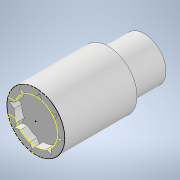
# Autodesk Inventor part: handle_base3
Saved by Autodesk Inventor 2021 (Build 250183000, 183)
## iProperties
Created: 2021-07-05
Part Number: handle_base3
Material: Generic
Document SubType Name: Modeling
Designer: teh18
Density: 1 g/cm^3
Appearance: Default
Author: teh18
Autodesk Inventor part; units mm, degrees
ref_plane "YZ Plane" through (0, 0, 0) normal (1, 0, 0) x (0, 1, 0)
ref_plane "XZ Plane" through (0, 0, 0) normal (0, 1, 0) x (-1, 0, 0)
ref_plane "XY Plane" through (0, 0, 0) normal (0, 0, 1) x (1, 0, 0)
sketch "Sketch1" plane through (0, 0, 0) normal (0, 0, 1) x (1, 0, 0)
  circle A0 centre (0, 0) radius 6
  circle A1 centre (0, 0) radius 20 projected
  circle A2 centre (0, 0) radius 5 projected
  arc A3 (6.0947, -0.2544) -> (5.2397, 3.1233) centre (0, 0) ccw projected
  arc A4 (4.1297, -4.4895) -> (5.9136, -1.4965) centre (0, 0) ccw projected
  arc A5 (-0.2544, -6.0947) -> (3.1233, -5.2397) centre (0, 0) ccw projected
  arc A6 (-4.4895, -4.1297) -> (-1.4965, -5.9136) centre (0, 0) ccw projected
  arc A7 (-6.0947, 0.2544) -> (-5.2397, -3.1233) centre (0, 0) ccw projected
  arc A8 (-4.1297, 4.4895) -> (-5.9136, 1.4965) centre (0, 0) ccw projected
  arc A9 (0.2544, 6.0947) -> (-3.1233, 5.2397) centre (0, 0) ccw projected
  arc A10 (4.4895, 4.1297) -> (1.4965, 5.9136) centre (0, 0) ccw projected
  line L0 (5.7362, 4.2762) -> (5.2397, 3.1233) projected
  line L1 (6.0947, -0.2544) -> (7.0798, -1.0323) projected
  line L2 (7.0798, -1.0323) -> (5.9136, -1.4965) projected
  line L3 (4.1297, -4.4895) -> (4.2762, -5.7362) projected
  line L4 (4.2762, -5.7362) -> (3.1233, -5.2397) projected
  line L5 (-0.2544, -6.0947) -> (-1.0323, -7.0798) projected
  line L6 (-1.0323, -7.0798) -> (-1.4965, -5.9136) projected
  line L7 (-4.4895, -4.1297) -> (-5.7362, -4.2762) projected
  line L8 (-5.7362, -4.2762) -> (-5.2397, -3.1233) projected
  line L9 (-6.0947, 0.2544) -> (-7.0798, 1.0323) projected
  line L10 (-7.0798, 1.0323) -> (-5.9136, 1.4965) projected
  line L11 (-4.1297, 4.4895) -> (-4.2762, 5.7362) projected
  line L12 (-4.2762, 5.7362) -> (-3.1233, 5.2397) projected
  line L13 (0.2544, 6.0947) -> (1.0323, 7.0798) projected
  line L14 (1.0323, 7.0798) -> (1.4965, 5.9136) projected
  line L15 (4.4895, 4.1297) -> (5.7362, 4.2762) projected
  line L16 (4.1567, -5.5758) -> (4.0244, -4.4502)
  arc A11 (4.0244, -4.4502) -> (5.8289, -1.4226) centre (0, 0) ccw
  line L17 (5.8289, -1.4226) -> (6.8819, -1.0035)
  line L18 (6.8819, -1.0035) -> (5.9924, -0.3011)
  arc A12 (5.9924, -0.3011) -> (5.1276, 3.1157) centre (0, 0) ccw
  line L19 (5.1276, 3.1157) -> (5.5758, 4.1567)
  line L20 (5.5758, 4.1567) -> (4.4502, 4.0244)
  arc A13 (4.4502, 4.0244) -> (1.4226, 5.8289) centre (0, 0) ccw
  line L21 (1.4226, 5.8289) -> (1.0035, 6.8819)
  line L22 (1.0035, 6.8819) -> (0.3011, 5.9924)
  arc A14 (0.3011, 5.9924) -> (-3.1157, 5.1276) centre (0, 0) ccw
  line L23 (-3.1157, 5.1276) -> (-4.1567, 5.5758)
  line L24 (-4.1567, 5.5758) -> (-4.0244, 4.4502)
  arc A15 (-4.0244, 4.4502) -> (-5.8289, 1.4226) centre (0, 0) ccw
  line L25 (-5.8289, 1.4226) -> (-6.8819, 1.0035)
  line L26 (-6.8819, 1.0035) -> (-5.9924, 0.3011)
  arc A16 (-5.9924, 0.3011) -> (-5.1276, -3.1157) centre (0, 0) ccw
  line L27 (-5.1276, -3.1157) -> (-5.5758, -4.1567)
  line L28 (-5.5758, -4.1567) -> (-4.4502, -4.0244)
  arc A17 (-4.4502, -4.0244) -> (-1.4226, -5.8289) centre (0, 0) ccw
  line L29 (-1.4226, -5.8289) -> (-1.0035, -6.8819)
  line L30 (-1.0035, -6.8819) -> (-0.3011, -5.9924)
  arc A18 (-0.3011, -5.9924) -> (3.1157, -5.1276) centre (0, 0) ccw
  line L31 (3.1157, -5.1276) -> (4.1567, -5.5758)
  point P0 (0, 0)
  point P1 (0, 0)
  point P2 (5.8289, -1.4226)
  point P3 (3.1157, -5.1276)
  point P4 (-1.4226, -5.8289)
  point P5 (-5.1276, -3.1157)
  point P6 (-5.8289, 1.4226)
  point P7 (-3.1157, 5.1276)
  point P8 (1.4226, 5.8289)
  point P9 (5.1276, 3.1157)
  dimension "d0" = 0.1
  dimension "d14" = 0.1
  constraints: 32 end point, 16 point on circle, 9 centre point, 23 other
  measures "d0" radial gap between concentric circles of A3 A0
  measures "d14" distance between parallel lines of L3 L16
extrude "Extrusion1" add sketch "Sketch1" against normal blind 10 contours A0 | A0 L20 L19 | L18 L17 A0 | A0 L22 L21 | L16 L31 A0 | A0 L24 L23 | L30 L29 A0 | A0 L26 L25 | L28 L27 A0
sketch "Sketch2" plane through (0, 0, 0) normal (0, 0, 1) x (1, 0, 0)
  circle A0 centre (0, 0) radius 6.1 projected
  arc A1 (5.9924, -0.3011) -> (5.1276, 3.1157) centre (0, 0) ccw projected
  circle A2 centre (0, 0) radius 18
  circle A3 centre (0, 0) radius 20 projected
  point P0 (0, 0)
  constraints: 1 centre point
extrude "Extrusion2" add sketch "Sketch2" along normal blind 20 contours A0 | A2
sketch "Sketch6" plane through (0, 0, 20) normal (0, 0, 1) x (0, -1, 0)
  circle A0 centre (0, 0) radius 8 projected
  arc A1 (-4.2421, -4.1006) -> (-1.5887, -5.6821) centre (0, 0) ccw projected
  line L0 (-1.5887, -5.6821) -> (-1.0323, -7.0798) projected
  line L1 (-1.0323, -7.0798) -> (-0.1, -5.8992) projected
  arc A2 (-0.1, -5.8992) -> (2.8945, -5.1412) centre (0, 0) ccw projected
  line L2 (2.8945, -5.1412) -> (4.2762, -5.7362) projected
  line L3 (4.2762, -5.7362) -> (4.1006, -4.2421) projected
  arc A3 (4.1006, -4.2421) -> (5.6821, -1.5887) centre (0, 0) ccw projected
  line L4 (5.6821, -1.5887) -> (7.0798, -1.0323) projected
  line L5 (7.0798, -1.0323) -> (5.8992, -0.1) projected
  arc A4 (5.8992, -0.1) -> (5.1412, 2.8945) centre (0, 0) ccw projected
  line L6 (5.1412, 2.8945) -> (5.7362, 4.2762) projected
  line L7 (5.7362, 4.2762) -> (4.2421, 4.1006) projected
  arc A5 (4.2421, 4.1006) -> (1.5887, 5.6821) centre (0, 0) ccw projected
  line L8 (1.5887, 5.6821) -> (1.0323, 7.0798) projected
  line L9 (1.0323, 7.0798) -> (0.1, 5.8992) projected
  arc A6 (0.1, 5.8992) -> (-2.8945, 5.1412) centre (0, 0) ccw projected
  line L10 (-2.8945, 5.1412) -> (-4.2762, 5.7362) projected
  line L11 (-4.2762, 5.7362) -> (-4.1006, 4.2421) projected
  arc A7 (-4.1006, 4.2421) -> (-5.6821, 1.5887) centre (0, 0) ccw projected
  line L12 (-5.6821, 1.5887) -> (-7.0798, 1.0323) projected
  line L13 (-7.0798, 1.0323) -> (-5.8992, 0.1) projected
  arc A8 (-5.8992, 0.1) -> (-5.1412, -2.8945) centre (0, 0) ccw projected
  line L14 (-5.1412, -2.8945) -> (-5.7362, -4.2762) projected
  line L15 (-5.7362, -4.2762) -> (-4.2421, -4.1006) projected
  arc A9 (4.2796, 4.2066) -> (1.664, 5.7655) centre (0, 0) ccw
  line L16 (4.2796, 4.2066) -> (5.8979, 4.3968)
  line L17 (5.8979, 4.3968) -> (5.2535, 2.9002)
  arc A10 (6.0006, -0.0517) -> (5.2535, 2.9002) centre (0, 0) ccw
  line L18 (6.0006, -0.0517) -> (7.2794, -1.0614)
  line L19 (7.2794, -1.0614) -> (5.7655, -1.664)
  arc A11 (4.2066, -4.2796) -> (5.7655, -1.664) centre (0, 0) ccw
  line L20 (4.2066, -4.2796) -> (4.3968, -5.8979)
  line L21 (4.3968, -5.8979) -> (2.9002, -5.2535)
  arc A12 (-0.0517, -6.0006) -> (2.9002, -5.2535) centre (0, 0) ccw
  line L22 (-0.0517, -6.0006) -> (-1.0614, -7.2794)
  line L23 (-1.0614, -7.2794) -> (-1.664, -5.7655)
  arc A13 (-4.2796, -4.2066) -> (-1.664, -5.7655) centre (0, 0) ccw
  line L24 (-4.2796, -4.2066) -> (-5.8979, -4.3968)
  line L25 (-5.8979, -4.3968) -> (-5.2535, -2.9002)
  arc A14 (-6.0006, 0.0517) -> (-5.2535, -2.9002) centre (0, 0) ccw
  line L26 (-6.0006, 0.0517) -> (-7.2794, 1.0614)
  line L27 (-7.2794, 1.0614) -> (-5.7655, 1.664)
  arc A15 (-4.2066, 4.2796) -> (-5.7655, 1.664) centre (0, 0) ccw
  line L28 (-4.2066, 4.2796) -> (-4.3968, 5.8979)
  line L29 (-4.3968, 5.8979) -> (-2.9002, 5.2535)
  arc A16 (0.0517, 6.0006) -> (-2.9002, 5.2535) centre (0, 0) ccw
  line L30 (0.0517, 6.0006) -> (1.0614, 7.2794)
  line L31 (1.0614, 7.2794) -> (1.664, 5.7655)
  point P0 (0, 0)
  constraints: 32 end point, 16 point on circle, 8 centre point, 23 other
extrude "Extrusion5" cut sketch "Sketch6" against normal blind 2.1 contours L15 L14 A8 L13 L12 A7 L11 L10 A6 L9 L8 A5 L7 L6 A4 L5 L4 A3 L3 L2 A2 L1 L0 A1 | L16 L17 A10 L18 L19 A11 L20 L21 A12 L22 L23 A13 L24 L25 A14 L26 L27 A15 L28 L29 A16 L30 L31 A9
body "Solid1"
